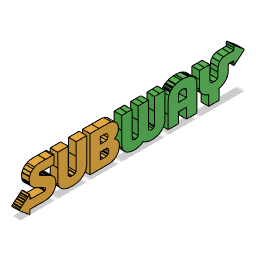
SUBWAY v0 (Autodesk Fusion 360 design; units mm, degrees)
Autodesk Fusion 360 part; units mm, degrees
note: some values were not read from the file. Set by a fixed rule: which sketch regions a step uses.
sketch "Sketch1" plane through (0, 0, 0) normal (1, 0, 0) x (0, 0, -1)
  spline S0 degree 3 poles (17.9669, -3.8504) (12.8198, -3.8249) (12.5225, -3.8587) (10.8168, -4.6775) knots 0 0 0 0 1 1 1 1
  spline S1 degree 3 poles (10.8168, -4.6775) (10.4326, -4.8619) (9.9837, -5.1092) (9.819, -5.2263) knots 0 0 0 0 1 1 1 1
  spline S2 degree 3 poles (9.819, -5.2263) (9.3261, -5.5771) (8.4224, -6.4653) (8.4224, -6.5991) knots 0 0 0 0 1 1 1 1
  spline S3 degree 3 poles (8.4224, -6.5991) (8.4224, -6.6674) (8.3955, -6.7231) (8.3627, -6.7231) knots 0 0 0 0 1 1 1 1
  spline S4 degree 3 poles (8.3627, -6.7231) (8.2047, -6.7231) (7.4935, -8.0577) (7.4922, -8.3563) knots 0 0 0 0 1 1 1 1
  spline S5 degree 3 poles (7.4922, -8.3563) (7.4918, -8.4679) (7.4655, -8.5874) (7.4341, -8.6222) knots 0 0 0 0 1 1 1 1
  spline S6 degree 3 poles (7.4341, -8.6222) (7.2242, -8.8543) (7.1579, -10.8776) (7.3318, -11.7452) knots 0 0 0 0 1 1 1 1
  spline S7 degree 3 poles (7.3318, -11.7452) (7.3904, -12.0379) (7.4649, -12.4116) (7.4977, -12.5762) knots 0 0 0 0 1 1 1 1
  spline S8 degree 3 poles (7.4977, -12.5762) (7.5599, -12.8888) (7.831, -13.454) (8.141, -13.9196) knots 0 0 0 0 1 1 1 1
  spline S9 degree 3 poles (8.141, -13.9196) (8.2411, -14.0697) (8.3527, -14.2401) (8.3891, -14.2986) knots 0 0 0 0 1 1 1 1
  spline S10 degree 3 poles (8.3891, -14.2986) (8.5537, -14.5634) (9.6552, -15.5795) (10.1208, -15.8954) knots 0 0 0 0 1 1 1 1
  spline S11 degree 3 poles (10.1208, -15.8954) (10.7697, -16.3356) (11.5575, -16.8141) (11.7594, -16.8915) knots 0 0 0 0 1 1 1 1
  spline S12 degree 3 poles (11.7594, -16.8915) (11.8446, -16.9241) (12.1837, -17.0969) (12.5129, -17.2752) knots 0 0 0 0 1 1 1 1
  spline S13 degree 3 poles (12.5129, -17.2752) (12.8421, -17.4534) (13.2458, -17.6552) (13.4105, -17.724) knots 0 0 0 0 1 1 1 1
  spline S14 degree 3 poles (13.4105, -17.724) (13.5751, -17.7928) (14.1293, -18.0504) (14.6414, -18.296) knots 0 0 0 0 1 1 1 1
  spline S15 degree 3 poles (14.6414, -18.296) (17.379, -19.6092) (17.6139, -19.7445) (17.8467, -20.1417) knots 0 0 0 0 1 1 1 1
  spline S16 degree 3 poles (17.8467, -20.1417) (18.0862, -20.5505) (18.0935, -20.9776) (17.8668, -21.3106) knots 0 0 0 0 1 1 1 1
  spline S17 degree 3 poles (17.8668, -21.3106) (17.7754, -21.4449) (17.6504, -21.5545) (17.5885, -21.5548) knots 0 0 0 0 1 1 1 1
  spline S18 degree 3 poles (17.5885, -21.5548) (17.5267, -21.555) (17.4543, -21.5906) (17.4281, -21.633) knots 0 0 0 0 1 1 1 1
  spline S19 degree 3 poles (17.4281, -21.633) (17.3789, -21.7122) (11.7353, -21.6755) (8.9377, -21.578) knots 0 0 0 0 1 1 1 1
  line L0 (8.9377, -21.578) -> (7.6905, -21.5346)
  line L1 (7.6905, -21.5346) -> (7.6905, -20.082)
  spline S20 degree 3 poles (7.6905, -20.082) (7.6905, -18.8349) (7.6762, -18.6286) (7.5905, -18.6286) knots 0 0 0 0 1 1 1 1
  spline S21 degree 3 poles (7.5905, -18.6286) (7.5357, -18.6286) (7.4913, -18.6586) (7.4913, -18.6952) knots 0 0 0 0 1 1 1 1
  spline S22 degree 3 poles (7.4913, -18.6952) (7.4913, -18.7318) (7.4571, -18.7619) (7.4153, -18.7619) knots 0 0 0 0 1 1 1 1
  spline S23 degree 3 poles (7.4153, -18.7619) (7.3328, -18.7619) (6.6268, -19.3372) (6.5402, -19.475) knots 0 0 0 0 1 1 1 1
  spline S24 degree 3 poles (6.5402, -19.475) (6.5109, -19.5216) (6.3962, -19.6068) (6.2852, -19.6642) knots 0 0 0 0 1 1 1 1
  spline S25 degree 3 poles (6.2852, -19.6642) (6.1742, -19.7216) (5.9129, -19.9253) (5.7054, -20.1161) knots 0 0 0 0 1 1 1 1
  spline S26 degree 3 poles (5.7054, -20.1161) (5.4978, -20.3069) (5.1889, -20.5586) (5.0186, -20.6758) knots 0 0 0 0 1 1 1 1
  spline S27 degree 3 poles (5.0186, -20.6758) (4.8483, -20.7929) (4.6992, -20.9123) (4.6868, -20.9409) knots 0 0 0 0 1 1 1 1
  spline S28 degree 3 poles (4.6868, -20.9409) (4.6532, -21.0188) (3.9986, -21.5555) (3.9372, -21.5555) knots 0 0 0 0 1 1 1 1
  spline S29 degree 3 poles (3.9372, -21.5555) (3.9079, -21.5555) (3.7899, -21.6549) (3.6752, -21.7765) knots 0 0 0 0 1 1 1 1
  spline S30 degree 3 poles (3.6752, -21.7765) (3.5602, -21.8987) (3.152, -22.2499) (2.7679, -22.5583) knots 0 0 0 0 1 1 1 1
  spline S31 degree 3 poles (2.7679, -22.5583) (2.3839, -22.8667) (2.0105, -23.179) (1.9378, -23.252) knots 0 0 0 0 1 1 1 1
  spline S32 degree 3 poles (1.9378, -23.252) (1.865, -23.3251) (1.6953, -23.4596) (1.561, -23.5513) knots 0 0 0 0 1 1 1 1
  spline S33 degree 3 poles (1.561, -23.5513) (1.4267, -23.6426) (1.1481, -23.8779) (0.9417, -24.0736) knots 0 0 0 0 1 1 1 1
  line L2 (0.9417, -24.0736) -> (0.5665, -24.4304)
  line L3 (0.5665, -24.4304) -> (0.9859, -24.8201)
  spline S34 degree 3 poles (0.9859, -24.8201) (1.2164, -25.0347) (1.4264, -25.2113) (1.4525, -25.2123) knots 0 0 0 0 1 1 1 1
  spline S35 degree 3 poles (1.4525, -25.2123) (1.4786, -25.2133) (1.7329, -25.4237) (2.0176, -25.6797) knots 0 0 0 0 1 1 1 1
  spline S36 degree 3 poles (2.0176, -25.6797) (2.3023, -25.9357) (2.5707, -26.1456) (2.6145, -26.1456) knots 0 0 0 0 1 1 1 1
  spline S37 degree 3 poles (2.6145, -26.1456) (2.6582, -26.1456) (2.7333, -26.1976) (2.7811, -26.2619) knots 0 0 0 0 1 1 1 1
  spline S38 degree 3 poles (2.7811, -26.2619) (2.8289, -26.3262) (3.0324, -26.5138) (3.233, -26.6782) knots 0 0 0 0 1 1 1 1
  spline S39 degree 3 poles (3.233, -26.6782) (3.4337, -26.8425) (3.6577, -27.0256) (3.7315, -27.0859) knots 0 0 0 0 1 1 1 1
  spline S40 degree 3 poles (3.7315, -27.0859) (3.8052, -27.1461) (4.0573, -27.3559) (4.2912, -27.5517) knots 0 0 0 0 1 1 1 1
  spline S41 degree 3 poles (4.2912, -27.5517) (4.525, -27.7475) (4.8442, -28.0037) (5.0004, -28.1207) knots 0 0 0 0 1 1 1 1
  spline S42 degree 3 poles (5.0004, -28.1207) (5.1566, -28.2376) (5.3877, -28.4367) (5.5143, -28.5633) knots 0 0 0 0 1 1 1 1
  spline S43 degree 3 poles (5.5143, -28.5633) (5.641, -28.6899) (5.8609, -28.8691) (6.0027, -28.9609) knots 0 0 0 0 1 1 1 1
  spline S44 degree 3 poles (6.0027, -28.9609) (6.1444, -29.0528) (6.4398, -29.2938) (6.6592, -29.4974) knots 0 0 0 0 1 1 1 1
  spline S45 degree 3 poles (6.6592, -29.4974) (6.8787, -29.7009) (7.0938, -29.8681) (7.1367, -29.8687) knots 0 0 0 0 1 1 1 1
  spline S46 degree 3 poles (7.1367, -29.8687) (7.1797, -29.8693) (7.2842, -29.9578) (7.3693, -30.0655) knots 0 0 0 0 1 1 1 1
  spline S47 degree 3 poles (7.3693, -30.0655) (7.6698, -30.446) (7.6865, -30.3812) (7.7057, -28.7555) knots 0 0 0 0 1 1 1 1
  line L4 (7.7057, -28.7555) -> (7.7235, -27.2425)
  line L5 (7.7235, -27.2425) -> (8.0227, -27.251)
  spline S48 degree 3 poles (8.0227, -27.251) (8.1873, -27.2553) (9.9156, -27.2648) (11.8635, -27.2727) knots 0 0 0 0 1 1 1 1
  spline S49 degree 3 poles (11.8635, -27.2727) (14.3296, -27.2827) (15.4052, -27.3091) (15.4052, -27.3587) knots 0 0 0 0 1 1 1 1
  spline S50 degree 3 poles (15.4052, -27.3587) (15.4052, -27.4401) (17.4754, -27.3847) (18.5314, -27.275) knots 0 0 0 0 1 1 1 1
  spline S51 degree 3 poles (18.5314, -27.275) (19.3597, -27.189) (20.4028, -26.9844) (20.5599, -26.8773) knots 0 0 0 0 1 1 1 1
  spline S52 degree 3 poles (20.5599, -26.8773) (20.5965, -26.8524) (20.8063, -26.7618) (21.0258, -26.6758) knots 0 0 0 0 1 1 1 1
  spline S53 degree 3 poles (21.0258, -26.6758) (21.2452, -26.5898) (21.44, -26.5011) (21.4583, -26.4789) knots 0 0 0 0 1 1 1 1
  spline S54 degree 3 poles (21.4583, -26.4789) (21.5226, -26.4008) (21.9988, -26.1448) (22.0799, -26.1448) knots 0 0 0 0 1 1 1 1
  spline S55 degree 3 poles (22.0799, -26.1448) (22.1251, -26.1448) (22.2664, -26.0482) (22.3939, -25.9293) knots 0 0 0 0 1 1 1 1
  spline S56 degree 3 poles (22.3939, -25.9293) (22.5214, -25.8104) (22.7399, -25.6228) (22.8799, -25.5131) knots 0 0 0 0 1 1 1 1
  spline S57 degree 3 poles (22.8799, -25.5131) (23.1681, -25.287) (23.8903, -24.3842) (24.1031, -23.9837) knots 0 0 0 0 1 1 1 1
  spline S58 degree 3 poles (24.1031, -23.9837) (24.3188, -23.5776) (24.6457, -22.5491) (24.7534, -21.9374) knots 0 0 0 0 1 1 1 1
  spline S59 degree 3 poles (24.7534, -21.9374) (24.969, -20.7123) (24.8306, -19.0957) (24.4255, -18.1027) knots 0 0 0 0 1 1 1 1
  spline S60 degree 3 poles (24.4255, -18.1027) (24.3297, -17.8678) (24.2511, -17.6501) (24.2511, -17.619) knots 0 0 0 0 1 1 1 1
  spline S61 degree 3 poles (24.2511, -17.619) (24.2511, -17.5505) (23.9224, -17.0259) (23.8209, -16.933) knots 0 0 0 0 1 1 1 1
  spline S62 degree 3 poles (23.8209, -16.933) (23.781, -16.8964) (23.6054, -16.68) (23.431, -16.4516) knots 0 0 0 0 1 1 1 1
  spline S63 degree 3 poles (23.431, -16.4516) (23.2566, -16.2233) (23.0527, -16.0038) (22.9783, -15.9641) knots 0 0 0 0 1 1 1 1
  spline S64 degree 3 poles (22.9783, -15.9641) (22.8475, -15.8941) (22.7341, -15.8017) (22.3094, -15.4238) knots 0 0 0 0 1 1 1 1
  spline S65 degree 3 poles (22.3094, -15.4238) (22.1989, -15.3254) (21.9991, -15.1942) (21.866, -15.1316) knots 0 0 0 0 1 1 1 1
  spline S66 degree 3 poles (21.866, -15.1316) (21.7329, -15.0689) (21.5204, -14.9319) (21.3932, -14.8277) knots 0 0 0 0 1 1 1 1
  spline S67 degree 3 poles (21.3932, -14.8277) (21.266, -14.7235) (21.1376, -14.6386) (21.1079, -14.6386) knots 0 0 0 0 1 1 1 1
  spline S68 degree 3 poles (21.1079, -14.6386) (21.0782, -14.6386) (20.8981, -14.5341) (20.708, -14.406) knots 0 0 0 0 1 1 1 1
  spline S69 degree 3 poles (20.708, -14.406) (20.5178, -14.278) (20.3211, -14.1727) (20.2708, -14.1727) knots 0 0 0 0 1 1 1 1
  spline S70 degree 3 poles (20.2708, -14.1727) (20.1639, -14.1727) (19.639, -13.8972) (19.6065, -13.8239) knots 0 0 0 0 1 1 1 1
  spline S71 degree 3 poles (19.6065, -13.8239) (19.5943, -13.7965) (19.542, -13.7743) (19.4902, -13.7743) knots 0 0 0 0 1 1 1 1
  spline S72 degree 3 poles (19.4902, -13.7743) (19.4384, -13.7743) (19.3964, -13.7442) (19.3964, -13.7076) knots 0 0 0 0 1 1 1 1
  spline S73 degree 3 poles (19.3964, -13.7076) (19.3964, -13.6711) (19.3473, -13.641) (19.2879, -13.641) knots 0 0 0 0 1 1 1 1
  spline S74 degree 3 poles (19.2879, -13.641) (19.2285, -13.641) (19.0116, -13.5562) (18.8058, -13.4526) knots 0 0 0 0 1 1 1 1
  spline S75 degree 3 poles (18.8058, -13.4526) (17.7171, -12.9047) (17.1625, -12.6389) (17.112, -12.641) knots 0 0 0 0 1 1 1 1
  spline S76 degree 3 poles (17.112, -12.641) (17.0811, -12.6424) (16.9742, -12.5854) (16.8749, -12.5147) knots 0 0 0 0 1 1 1 1
  spline S77 degree 3 poles (16.8749, -12.5147) (16.7755, -12.444) (16.6064, -12.3648) (16.4989, -12.3387) knots 0 0 0 0 1 1 1 1
  spline S78 degree 3 poles (16.4989, -12.3387) (16.3914, -12.3127) (15.9966, -12.1236) (15.6215, -11.9186) knots 0 0 0 0 1 1 1 1
  spline S79 degree 3 poles (15.6215, -11.9186) (15.2463, -11.7136) (14.8125, -11.4808) (14.6572, -11.4016) knots 0 0 0 0 1 1 1 1
  spline S80 degree 3 poles (14.6572, -11.4016) (14.5019, -11.3224) (14.2863, -11.1648) (14.1781, -11.0512) knots 0 0 0 0 1 1 1 1
  spline S81 degree 3 poles (14.1781, -11.0512) (13.9981, -10.8621) (13.9813, -10.8048) (13.9813, -10.3707) knots 0 0 0 0 1 1 1 1
  spline S82 degree 3 poles (13.9813, -10.3707) (13.9813, -9.9158) (13.9901, -9.8891) (14.2006, -9.7134) knots 0 0 0 0 1 1 1 1
  spline S83 degree 3 poles (14.2006, -9.7134) (14.3213, -9.6126) (14.5146, -9.5167) (14.63, -9.4994) knots 0 0 0 0 1 1 1 1
  spline S84 degree 3 poles (14.63, -9.4994) (14.7455, -9.4821) (16.8154, -9.4834) (19.2298, -9.5025) knots 0 0 0 0 1 1 1 1
  line L6 (19.2298, -9.5025) -> (23.6197, -9.5374)
  line L7 (23.6197, -9.5374) -> (23.6073, -6.75)
  line L8 (23.6073, -6.75) -> (23.5941, -3.9633)
  line L9 (23.5941, -3.9633) -> (22.8089, -3.9176)
  spline S85 degree 3 poles (22.8089, -3.9176) (22.3759, -3.8926) (20.1966, -3.8625) (17.9654, -3.8514) knots 0 0 0 0 1 1 1 1
  line L10 (17.9654, -3.8514) -> (17.9669, -3.8504)
  line L11 (26.1112, -3.8636) -> (26.1336, -12.8925)
  spline S86 degree 3 poles (26.1336, -12.8925) (26.1532, -20.9268) (26.1673, -21.9579) (26.2615, -22.254) knots 0 0 0 0 1 1 1 1
  spline S87 degree 3 poles (26.2615, -22.254) (26.459, -22.8741) (26.666, -23.3788) (26.8561, -23.7012) knots 0 0 0 0 1 1 1 1
  spline S88 degree 3 poles (26.8561, -23.7012) (26.9602, -23.8779) (27.046, -24.0519) (27.046, -24.088) knots 0 0 0 0 1 1 1 1
  spline S89 degree 3 poles (27.046, -24.088) (27.046, -24.3202) (28.785, -26.1452) (29.0063, -26.1452) knots 0 0 0 0 1 1 1 1
  spline S90 degree 3 poles (29.0063, -26.1452) (29.0305, -26.1452) (29.176, -26.2275) (29.3296, -26.3281) knots 0 0 0 0 1 1 1 1
  spline S91 degree 3 poles (29.3296, -26.3281) (30.0784, -26.8188) (30.3659, -26.9586) (31.1798, -27.2304) knots 0 0 0 0 1 1 1 1
  spline S92 degree 3 poles (31.1798, -27.2304) (32.073, -27.5287) (32.8887, -27.7261) (33.6967, -27.8389) knots 0 0 0 0 1 1 1 1
  spline S93 degree 3 poles (33.6967, -27.8389) (34.5621, -27.9597) (36.694, -27.961) (37.488, -27.8412) knots 0 0 0 0 1 1 1 1
  spline S94 degree 3 poles (37.488, -27.8412) (38.6521, -27.6656) (39.5088, -27.4479) (40.125, -27.1707) knots 0 0 0 0 1 1 1 1
  spline S95 degree 3 poles (40.125, -27.1707) (40.2403, -27.1188) (40.3853, -27.0761) (40.4467, -27.0761) knots 0 0 0 0 1 1 1 1
  spline S96 degree 3 poles (40.4467, -27.0761) (40.5792, -27.0761) (41.6532, -26.5137) (41.8443, -26.3444) knots 0 0 0 0 1 1 1 1
  spline S97 degree 3 poles (41.8443, -26.3444) (41.9174, -26.2796) (42.0873, -26.1708) (42.221, -26.1025) knots 0 0 0 0 1 1 1 1
  spline S98 degree 3 poles (42.221, -26.1025) (42.5395, -25.94) (43.6561, -24.904) (43.7883, -24.6483) knots 0 0 0 0 1 1 1 1
  spline S99 degree 3 poles (43.7883, -24.6483) (43.8451, -24.5386) (43.9561, -24.3839) (44.0348, -24.3042) knots 0 0 0 0 1 1 1 1
  spline S100 degree 3 poles (44.0348, -24.3042) (44.2262, -24.1106) (44.6826, -23.2713) (44.7829, -22.9283) knots 0 0 0 0 1 1 1 1
  spline S101 degree 3 poles (44.7829, -22.9283) (44.8271, -22.777) (44.9385, -22.3839) (45.0309, -22.0547) knots 0 0 0 0 1 1 1 1
  line L12 (45.0309, -22.0547) -> (45.1991, -21.4555)
  line L13 (45.1991, -21.4555) -> (45.2015, -12.6599)
  line L14 (45.2015, -12.6599) -> (45.2039, -3.8636)
  line L15 (45.2039, -3.8636) -> (41.7119, -3.8636)
  line L16 (41.7119, -3.8636) -> (38.2198, -3.8636)
  line L17 (38.2198, -3.8636) -> (38.2198, -12.2726)
  spline S102 degree 3 poles (38.2198, -12.2726) (38.2198, -17.4562) (38.1954, -20.7467) (38.1563, -20.8495) knots 0 0 0 0 1 1 1 1
  spline S103 degree 3 poles (38.1563, -20.8495) (38.0741, -21.0656) (37.6314, -21.5556) (37.5183, -21.5556) knots 0 0 0 0 1 1 1 1
  spline S104 degree 3 poles (37.5183, -21.5556) (37.4703, -21.5556) (37.3908, -21.5956) (37.3416, -21.6448) knots 0 0 0 0 1 1 1 1
  spline S105 degree 3 poles (37.3416, -21.6448) (37.1097, -21.8767) (36.5438, -21.9881) (35.5929, -21.9881) knots 0 0 0 0 1 1 1 1
  line L18 (35.5929, -21.9881) -> (34.6619, -21.9881)
  line L19 (34.6619, -21.9881) -> (34.1341, -21.7316)
  spline S106 degree 3 poles (34.1341, -21.7316) (33.5796, -21.4633) (33.4268, -21.3192) (33.1796, -20.8307) knots 0 0 0 0 1 1 1 1
  line L20 (33.1796, -20.8307) -> (33.03, -20.5353)
  line L21 (33.03, -20.5353) -> (33.03, -12.1994)
  line L22 (33.03, -12.1994) -> (33.03, -3.8634)
  line L23 (33.03, -3.8634) -> (29.5697, -3.8634)
  line L24 (29.5697, -3.8634) -> (26.1094, -3.8634)
  line L25 (26.1094, -3.8634) -> (26.1112, -3.8636)
  line L26 (47.3975, -3.8643) -> (47.3975, -15.6364)
  line L27 (47.3975, -15.6364) -> (47.3975, -27.4093)
  line L28 (47.3975, -27.4093) -> (53.6662, -27.407)
  spline S107 degree 3 poles (53.6662, -27.407) (60.04, -27.4049) (60.6452, -27.3851) (61.4306, -27.1473) knots 0 0 0 0 1 1 1 1
  spline S108 degree 3 poles (61.4306, -27.1473) (61.5584, -27.1087) (61.7446, -27.0768) (61.8446, -27.0768) knots 0 0 0 0 1 1 1 1
  spline S109 degree 3 poles (61.8446, -27.0768) (62.0206, -27.0768) (62.6478, -26.8233) (63.1933, -26.5319) knots 0 0 0 0 1 1 1 1
  spline S110 degree 3 poles (63.1933, -26.5319) (63.3397, -26.4537) (63.6234, -26.3022) (63.8235, -26.1955) knots 0 0 0 0 1 1 1 1
  spline S111 degree 3 poles (63.8235, -26.1955) (64.1353, -26.0291) (64.516, -25.7092) (65.1165, -25.1095) knots 0 0 0 0 1 1 1 1
  spline S112 degree 3 poles (65.1165, -25.1095) (65.2974, -24.9288) (65.7039, -24.3619) (65.9094, -24.0026) knots 0 0 0 0 1 1 1 1
  spline S113 degree 3 poles (65.9094, -24.0026) (66.0869, -23.6924) (66.489, -22.5389) (66.6233, -21.9554) knots 0 0 0 0 1 1 1 1
  spline S114 degree 3 poles (66.6233, -21.9554) (66.7371, -21.4609) (66.7969, -20.173) (66.7342, -19.561) knots 0 0 0 0 1 1 1 1
  spline S115 degree 3 poles (66.7342, -19.561) (66.6863, -19.0933) (66.4022, -18.0126) (66.2885, -17.865) knots 0 0 0 0 1 1 1 1
  spline S116 degree 3 poles (66.2885, -17.865) (66.2603, -17.8284) (66.199, -17.6788) (66.1528, -17.5324) knots 0 0 0 0 1 1 1 1
  spline S117 degree 3 poles (66.1528, -17.5324) (66.0268, -17.1328) (65.2329, -16.1727) (64.6661, -15.7349) knots 0 0 0 0 1 1 1 1
  spline S118 degree 3 poles (64.6661, -15.7349) (64.525, -15.6259) (64.3394, -15.4727) (64.2537, -15.3938) knots 0 0 0 0 1 1 1 1
  spline S119 degree 3 poles (64.2537, -15.3938) (64.168, -15.315) (63.9771, -15.1972) (63.8289, -15.1318) knots 0 0 0 0 1 1 1 1
  spline S120 degree 3 poles (63.8289, -15.1318) (63.6807, -15.0664) (63.5592, -14.994) (63.5592, -14.9714) knots 0 0 0 0 1 1 1 1
  spline S121 degree 3 poles (63.5592, -14.9714) (63.5592, -14.9304) (63.9281, -14.6388) (63.9801, -14.6388) knots 0 0 0 0 1 1 1 1
  spline S122 degree 3 poles (63.9801, -14.6388) (64.0297, -14.6388) (65.0893, -13.5925) (65.0893, -13.5435) knots 0 0 0 0 1 1 1 1
  spline S123 degree 3 poles (65.0893, -13.5435) (65.0893, -13.5171) (65.1453, -13.4158) (65.2141, -13.3187) knots 0 0 0 0 1 1 1 1
  spline S124 degree 3 poles (65.2141, -13.3187) (65.4108, -13.0414) (65.7945, -12.293) (65.8869, -12.0064) knots 0 0 0 0 1 1 1 1
  spline S125 degree 3 poles (65.8869, -12.0064) (65.9332, -11.8631) (66.0049, -11.7035) (66.0459, -11.6522) knots 0 0 0 0 1 1 1 1
  spline S126 degree 3 poles (66.0459, -11.6522) (66.0954, -11.5901) (66.118, -11.1331) (66.1148, -10.2887) knots 0 0 0 0 1 1 1 1
  spline S127 degree 3 poles (66.1148, -10.2887) (66.1103, -9.1063) (66.0981, -8.9805) (65.9342, -8.4648) knots 0 0 0 0 1 1 1 1
  spline S128 degree 3 poles (65.9342, -8.4648) (65.7321, -7.8289) (65.2664, -6.8576) (65.0226, -6.5634) knots 0 0 0 0 1 1 1 1
  spline S129 degree 3 poles (65.0226, -6.5634) (64.5939, -6.0458) (64.0884, -5.5515) (63.7096, -5.2805) knots 0 0 0 0 1 1 1 1
  spline S130 degree 3 poles (63.7096, -5.2805) (63.1831, -4.904) (62.2596, -4.4536) (61.5647, -4.2341) knots 0 0 0 0 1 1 1 1
  spline S131 degree 3 poles (61.5647, -4.2341) (60.4932, -3.8963) (59.7708, -3.8643) (53.3097, -3.8643) knots 0 0 0 0 1 1 1 1
  line L29 (53.3097, -3.8643) -> (47.3971, -3.8643)
  line L30 (47.3971, -3.8643) -> (47.3975, -3.8643)
  line L31 (54.2484, -8.9765) -> (56.1274, -8.9982)
  spline S132 degree 3 poles (56.1274, -8.9982) (58.1657, -9.0212) (58.1504, -9.0188) (58.6326, -9.4245) knots 0 0 0 0 1 1 1 1
  spline S133 degree 3 poles (58.6326, -9.4245) (59.1501, -9.86) (59.3525, -10.864) (59.1334, -11.9127) knots 0 0 0 0 1 1 1 1
  spline S134 degree 3 poles (59.1334, -11.9127) (59.0568, -12.2793) (58.6065, -12.8887) (58.2861, -13.0599) knots 0 0 0 0 1 1 1 1
  spline S135 degree 3 poles (58.2861, -13.0599) (58.0176, -13.2035) (57.9279, -13.2101) (56.1274, -13.2305) knots 0 0 0 0 1 1 1 1
  line L32 (56.1274, -13.2305) -> (54.2484, -13.2522)
  line L33 (54.2484, -13.2522) -> (54.2484, -11.1143)
  line L34 (54.2484, -11.1143) -> (54.2484, -8.9765)
  spline S136 degree 3 poles (54.298, -17.7526) (54.3255, -17.7413) (55.3082, -17.7467) (56.4816, -17.765) knots 0 0 0 0 1 1 1 1
  line L35 (56.4816, -17.765) -> (58.6148, -17.7983)
  line L36 (58.6148, -17.7983) -> (58.8946, -17.9836)
  spline S137 degree 3 poles (58.8946, -17.9836) (59.0487, -18.0856) (59.2857, -18.3405) (59.421, -18.5494) knots 0 0 0 0 1 1 1 1
  line L37 (59.421, -18.5494) -> (59.6667, -18.9293)
  line L38 (59.6667, -18.9293) -> (59.6675, -19.899)
  spline S138 degree 3 poles (59.6675, -19.899) (59.6683, -20.7868) (59.6553, -20.897) (59.5078, -21.2121) knots 0 0 0 0 1 1 1 1
  spline S139 degree 3 poles (59.5078, -21.2121) (59.4193, -21.4014) (59.3064, -21.5563) (59.2567, -21.5563) knots 0 0 0 0 1 1 1 1
  spline S140 degree 3 poles (59.2567, -21.5563) (59.2069, -21.5563) (59.1494, -21.599) (59.1295, -21.6508) knots 0 0 0 0 1 1 1 1
  spline S141 degree 3 poles (59.1295, -21.6508) (59.0721, -21.8004) (58.6328, -22.059) (58.2924, -22.1438) knots 0 0 0 0 1 1 1 1
  spline S142 degree 3 poles (58.2924, -22.1438) (58.0914, -22.1939) (57.3155, -22.2213) (56.1142, -22.2213) knots 0 0 0 0 1 1 1 1
  line L39 (56.1142, -22.2213) -> (54.2484, -22.2213)
  line L40 (54.2484, -22.2213) -> (54.2484, -19.9974)
  spline S143 degree 3 poles (54.2484, -19.9974) (54.2484, -18.7741) (54.2706, -17.7639) (54.298, -17.7526) knots 0 0 0 0 1 1 1 1
  spline S144 degree 3 poles (142.434, -0.8661) (142.3862, -0.8922) (142.3825, -1.191) (142.3813, -2.2505) knots 0 0 0 0 1 1 1 1
  line L41 (142.3813, -2.2505) -> (142.3797, -3.7302)
  line L42 (142.3797, -3.7302) -> (139.7032, -3.7318)
  spline S145 degree 3 poles (139.7032, -3.7318) (137.1275, -3.7331) (136.7848, -3.7522) (135.6459, -3.9558) knots 0 0 0 0 1 1 1 1
  spline S146 degree 3 poles (135.6459, -3.9558) (134.7048, -4.1241) (133.6691, -4.7468) (133.0438, -5.5209) knots 0 0 0 0 1 1 1 1
  spline S147 degree 3 poles (133.0438, -5.5209) (132.5335, -6.1524) (132.2214, -6.8603) (131.9702, -7.9541) knots 0 0 0 0 1 1 1 1
  spline S148 degree 3 poles (131.9702, -7.9541) (131.945, -8.0638) (131.9049, -9.3804) (131.881, -10.8802) knots 0 0 0 0 1 1 1 1
  spline S149 degree 3 poles (131.881, -10.8802) (131.8332, -13.8832) (131.8538, -13.7377) (131.3888, -14.3164) knots 0 0 0 0 1 1 1 1
  spline S150 degree 3 poles (131.3888, -14.3164) (131.012, -14.7855) (130.0923, -15.1032) (129.1107, -15.1032) knots 0 0 0 0 1 1 1 1
  spline S151 degree 3 poles (129.1107, -15.1032) (128.6308, -15.1032) (127.7928, -14.9093) (127.5077, -14.7327) knots 0 0 0 0 1 1 1 1
  spline S152 degree 3 poles (127.5077, -14.7327) (127.1453, -14.5083) (126.7397, -14.102) (126.6612, -13.8847) knots 0 0 0 0 1 1 1 1
  spline S153 degree 3 poles (126.6612, -13.8847) (126.6079, -13.7371) (126.575, -12.2087) (126.5511, -8.7848) knots 0 0 0 0 1 1 1 1
  line L43 (126.5511, -8.7848) -> (126.517, -3.8969)
  line L44 (126.517, -3.8969) -> (123.1079, -3.8799)
  line L45 (123.1079, -3.8799) -> (119.6996, -3.862)
  line L46 (119.6996, -3.862) -> (119.7004, -9.0671)
  spline S154 degree 3 poles (119.7004, -9.0671) (119.7012, -11.9299) (119.729, -14.4618) (119.7624, -14.6932) knots 0 0 0 0 1 1 1 1
  spline S155 degree 3 poles (119.7624, -14.6932) (119.8358, -15.2002) (120.1152, -16.144) (120.3275, -16.6008) knots 0 0 0 0 1 1 1 1
  spline S156 degree 3 poles (120.3275, -16.6008) (120.7281, -17.4629) (121.6691, -18.5402) (122.5336, -19.1278) knots 0 0 0 0 1 1 1 1
  spline S157 degree 3 poles (122.5336, -19.1278) (122.7489, -19.2741) (122.9843, -19.4476) (123.0568, -19.513) knots 0 0 0 0 1 1 1 1
  spline S158 degree 3 poles (123.0568, -19.513) (123.1293, -19.5784) (123.2638, -19.6492) (123.356, -19.6704) knots 0 0 0 0 1 1 1 1
  spline S159 degree 3 poles (123.356, -19.6704) (123.4482, -19.6916) (123.6455, -19.7783) (123.7948, -19.8634) knots 0 0 0 0 1 1 1 1
  spline S160 degree 3 poles (123.7948, -19.8634) (124.1062, -20.0408) (124.9715, -20.3949) (125.4358, -20.5346) knots 0 0 0 0 1 1 1 1
  line L47 (125.4358, -20.5346) -> (125.752, -20.63)
  line L48 (125.752, -20.63) -> (125.752, -24.0189)
  line L49 (125.752, -24.0189) -> (125.752, -27.4087)
  line L50 (125.752, -27.4087) -> (129.2107, -27.4087)
  line L51 (129.2107, -27.4087) -> (132.6694, -27.4087)
  line L52 (132.6694, -27.4087) -> (132.6694, -24.0321)
  line L53 (132.6694, -24.0321) -> (132.6694, -20.6556)
  line L54 (132.6694, -20.6556) -> (133.2182, -20.4657)
  spline S161 degree 3 poles (133.2182, -20.4657) (134.0185, -20.1889) (135.572, -19.4134) (135.9901, -19.082) knots 0 0 0 0 1 1 1 1
  spline S162 degree 3 poles (135.9901, -19.082) (136.5198, -18.6623) (137.3717, -17.7807) (137.6172, -17.3984) knots 0 0 0 0 1 1 1 1
  spline S163 degree 3 poles (137.6172, -17.3984) (137.9206, -16.9259) (138.3516, -15.944) (138.4784, -15.4365) knots 0 0 0 0 1 1 1 1
  spline S164 degree 3 poles (138.4784, -15.4365) (138.6593, -14.7121) (138.7198, -13.8269) (138.7217, -11.8453) knots 0 0 0 0 1 1 1 1
  spline S165 degree 3 poles (138.7217, -11.8453) (138.7229, -10.8027) (138.7416, -9.8824) (138.7636, -9.8005) knots 0 0 0 0 1 1 1 1
  spline S166 degree 3 poles (138.7636, -9.8005) (138.8286, -9.5579) (139.1739, -9.5127) (140.8286, -9.5323) knots 0 0 0 0 1 1 1 1
  line L55 (140.8286, -9.5323) -> (142.3463, -9.5501)
  line L56 (142.3463, -9.5501) -> (142.3649, -10.9973)
  spline S167 degree 3 poles (142.3649, -10.9973) (142.376, -11.886) (142.4078, -12.4437) (142.4479, -12.4437) knots 0 0 0 0 1 1 1 1
  spline S168 degree 3 poles (142.4479, -12.4437) (142.4837, -12.4437) (142.513, -12.4136) (142.513, -12.377) knots 0 0 0 0 1 1 1 1
  spline S169 degree 3 poles (142.513, -12.377) (142.513, -12.3405) (142.5502, -12.3105) (142.5959, -12.3104) knots 0 0 0 0 1 1 1 1
  spline S170 degree 3 poles (142.5959, -12.3104) (142.6417, -12.3102) (142.9087, -12.1004) (143.1889, -11.8445) knots 0 0 0 0 1 1 1 1
  spline S171 degree 3 poles (143.1889, -11.8445) (143.4692, -11.5886) (143.7239, -11.3794) (143.7555, -11.3794) knots 0 0 0 0 1 1 1 1
  spline S172 degree 3 poles (143.7555, -11.3794) (143.7871, -11.3794) (143.9918, -11.2104) (144.2097, -11.0042) knots 0 0 0 0 1 1 1 1
  spline S173 degree 3 poles (144.2097, -11.0042) (144.4277, -10.7981) (144.7113, -10.5615) (144.8399, -10.4779) knots 0 0 0 0 1 1 1 1
  spline S174 degree 3 poles (144.8399, -10.4779) (144.9686, -10.3944) (145.253, -10.159) (145.4725, -9.9555) knots 0 0 0 0 1 1 1 1
  spline S175 degree 3 poles (145.4725, -9.9555) (145.692, -9.7519) (145.8942, -9.5855) (145.9213, -9.5849) knots 0 0 0 0 1 1 1 1
  spline S176 degree 3 poles (145.9213, -9.5849) (145.9484, -9.5844) (146.1297, -9.4417) (146.3244, -9.2679) knots 0 0 0 0 1 1 1 1
  spline S177 degree 3 poles (146.3244, -9.2679) (146.7573, -8.8814) (148.023, -7.8299) (148.394, -7.5486) knots 0 0 0 0 1 1 1 1
  spline S178 degree 3 poles (148.394, -7.5486) (148.5433, -7.4354) (148.83, -7.1874) (149.0312, -6.9975) knots 0 0 0 0 1 1 1 1
  line L57 (149.0312, -6.9975) -> (149.397, -6.6518)
  line L58 (149.397, -6.6518) -> (148.9405, -6.2224)
  spline S179 degree 3 poles (148.9405, -6.2224) (148.6894, -5.9859) (148.4444, -5.7922) (148.3963, -5.7922) knots 0 0 0 0 1 1 1 1
  spline S180 degree 3 poles (148.3963, -5.7922) (148.3483, -5.7922) (148.2545, -5.7241) (148.1878, -5.641) knots 0 0 0 0 1 1 1 1
  spline S181 degree 3 poles (148.1878, -5.641) (148.1211, -5.5579) (147.8872, -5.3489) (147.6677, -5.1759) knots 0 0 0 0 1 1 1 1
  spline S182 degree 3 poles (147.6677, -5.1759) (147.4482, -5.003) (147.2084, -4.8056) (147.1352, -4.7372) knots 0 0 0 0 1 1 1 1
  spline S183 degree 3 poles (147.1352, -4.7372) (147.062, -4.6688) (146.6816, -4.3531) (146.2895, -4.0357) knots 0 0 0 0 1 1 1 1
  spline S184 degree 3 poles (146.2895, -4.0357) (145.8974, -3.7182) (145.4883, -3.3701) (145.3803, -3.2621) knots 0 0 0 0 1 1 1 1
  spline S185 degree 3 poles (145.3803, -3.2621) (145.2722, -3.154) (145.157, -3.0652) (145.1245, -3.0652) knots 0 0 0 0 1 1 1 1
  spline S186 degree 3 poles (145.1245, -3.0652) (145.0919, -3.0652) (144.8381, -2.8562) (144.5601, -2.6001) knots 0 0 0 0 1 1 1 1
  spline S187 degree 3 poles (144.5601, -2.6001) (144.2823, -2.3452) (144.0244, -2.1354) (143.9926, -2.1354) knots 0 0 0 0 1 1 1 1
  spline S188 degree 3 poles (143.9926, -2.1354) (143.9586, -2.1354) (143.7538, -1.9692) (143.5376, -1.7656) knots 0 0 0 0 1 1 1 1
  spline S189 degree 3 poles (143.5376, -1.7656) (143.3214, -1.5621) (143.025, -1.3187) (142.8787, -1.2254) knots 0 0 0 0 1 1 1 1
  spline S190 degree 3 poles (142.8787, -1.2254) (142.7324, -1.1321) (142.5605, -0.9919) (142.4973, -0.9138) knots 0 0 0 0 1 1 1 1
  spline S191 degree 3 poles (142.4973, -0.9138) (142.4699, -0.8799) (142.4497, -0.8585) (142.4338, -0.8672) knots 0 0 0 0 1 1 1 1
  line L59 (142.4338, -0.8672) -> (142.434, -0.8661)
  spline S192 degree 3 poles (108.6973, -3.1613) (108.2854, -3.1547) (107.8754, -3.1666) (107.4756, -3.1977) knots 0 0 0 0 1 1 1 1
  spline S193 degree 3 poles (107.4756, -3.1977) (106.1692, -3.2995) (104.8711, -3.5671) (104.1208, -3.8899) knots 0 0 0 0 1 1 1 1
  spline S194 degree 3 poles (104.1208, -3.8899) (103.9848, -3.9484) (103.8228, -3.9969) (103.7604, -3.9969) knots 0 0 0 0 1 1 1 1
  spline S195 degree 3 poles (103.7604, -3.9969) (103.6164, -3.9969) (102.6676, -4.4828) (102.3186, -4.7356) knots 0 0 0 0 1 1 1 1
  spline S196 degree 3 poles (102.3186, -4.7356) (102.173, -4.8411) (102.0174, -4.9278) (101.9737, -4.9278) knots 0 0 0 0 1 1 1 1
  spline S197 degree 3 poles (101.9737, -4.9278) (101.9299, -4.9278) (101.7928, -5.0249) (101.6683, -5.1441) knots 0 0 0 0 1 1 1 1
  spline S198 degree 3 poles (101.6683, -5.1441) (101.5438, -5.2632) (101.2543, -5.5227) (101.0257, -5.72) knots 0 0 0 0 1 1 1 1
  spline S199 degree 3 poles (101.0257, -5.72) (100.797, -5.9173) (100.6102, -6.1073) (100.6102, -6.1425) knots 0 0 0 0 1 1 1 1
  spline S200 degree 3 poles (100.6102, -6.1425) (100.6102, -6.1777) (100.4952, -6.3449) (100.3544, -6.5146) knots 0 0 0 0 1 1 1 1
  spline S201 degree 3 poles (100.3544, -6.5146) (99.9248, -7.0323) (99.7634, -7.3253) (99.487, -8.0873) knots 0 0 0 0 1 1 1 1
  spline S202 degree 3 poles (99.487, -8.0873) (98.9898, -9.4582) (99.0142, -8.9124) (99.0142, -18.6696) knots 0 0 0 0 1 1 1 1
  line L60 (99.0142, -18.6696) -> (99.0142, -27.4088)
  line L61 (99.0142, -27.4088) -> (102.4396, -27.4088)
  line L62 (102.4396, -27.4088) -> (105.8642, -27.4088)
  line L63 (105.8642, -27.4088) -> (105.8642, -24.0168)
  line L64 (105.8642, -24.0168) -> (105.8642, -20.6247)
  line L65 (105.8642, -20.6247) -> (108.4919, -20.6247)
  line L66 (108.4919, -20.6247) -> (111.1189, -20.6247)
  line L67 (111.1189, -20.6247) -> (111.1189, -24.0168)
  line L68 (111.1189, -24.0168) -> (111.1189, -27.4088)
  line L69 (111.1189, -27.4088) -> (114.5443, -27.4088)
  line L70 (114.5443, -27.4088) -> (117.9696, -27.4088)
  line L71 (117.9696, -27.4088) -> (117.9696, -18.7125)
  spline S203 degree 3 poles (117.9696, -18.7125) (117.9695, -11.1679) (117.9557, -9.9384) (117.8665, -9.4284) knots 0 0 0 0 1 1 1 1
  spline S204 degree 3 poles (117.8665, -9.4284) (117.7078, -8.5209) (117.1613, -7.1123) (116.8449, -6.796) knots 0 0 0 0 1 1 1 1
  spline S205 degree 3 poles (116.8449, -6.796) (116.7772, -6.7283) (116.6006, -6.4944) (116.4527, -6.2766) knots 0 0 0 0 1 1 1 1
  spline S206 degree 3 poles (116.4527, -6.2766) (116.3048, -6.0589) (116.1132, -5.8344) (116.0264, -5.7775) knots 0 0 0 0 1 1 1 1
  spline S207 degree 3 poles (116.0264, -5.7775) (115.9395, -5.7206) (115.7073, -5.5212) (115.5109, -5.3349) knots 0 0 0 0 1 1 1 1
  spline S208 degree 3 poles (115.5109, -5.3349) (115.3145, -5.1485) (115.094, -4.9774) (115.021, -4.9543) knots 0 0 0 0 1 1 1 1
  spline S209 degree 3 poles (115.021, -4.9543) (114.948, -4.9311) (114.7516, -4.814) (114.5838, -4.6946) knots 0 0 0 0 1 1 1 1
  spline S210 degree 3 poles (114.5838, -4.6946) (114.1949, -4.4169) (113.5122, -4.0749) (113.1233, -3.9614) knots 0 0 0 0 1 1 1 1
  spline S211 degree 3 poles (113.1233, -3.9614) (112.9566, -3.9127) (112.5637, -3.7936) (112.2542, -3.697) knots 0 0 0 0 1 1 1 1
  spline S212 degree 3 poles (112.2542, -3.697) (111.1905, -3.367) (109.9364, -3.1812) (108.7021, -3.1614) knots 0 0 0 0 1 1 1 1
  line L72 (108.7021, -3.1614) -> (108.6973, -3.1613)
  line L73 (96.8902, -3.862) -> (93.4463, -3.8798)
  line L74 (93.4463, -3.8798) -> (90.0015, -3.8969)
  line L75 (90.0015, -3.8969) -> (89.9682, -12.3436)
  line L76 (89.9682, -12.3436) -> (89.9348, -20.7911)
  line L77 (89.9348, -20.7911) -> (89.7558, -21.0949)
  spline S213 degree 3 poles (89.7558, -21.0949) (89.5334, -21.4731) (89.496, -21.5032) (89.0039, -21.6871) knots 0 0 0 0 1 1 1 1
  spline S214 degree 3 poles (89.0039, -21.6871) (88.2185, -21.9807) (86.9259, -21.8388) (86.4568, -21.4073) knots 0 0 0 0 1 1 1 1
  spline S215 degree 3 poles (86.4568, -21.4073) (86.3666, -21.3244) (86.2375, -21.1366) (86.1699, -20.9903) knots 0 0 0 0 1 1 1 1
  spline S216 degree 3 poles (86.1699, -20.9903) (86.0526, -20.7362) (86.0475, -20.35) (86.0459, -12.3987) knots 0 0 0 0 1 1 1 1
  spline S217 degree 3 poles (86.0459, -12.3987) (86.0451, -7.82) (86.0263, -4.027) (86.0041, -3.9691) knots 0 0 0 0 1 1 1 1
  spline S218 degree 3 poles (86.0041, -3.9691) (85.968, -3.8751) (85.604, -3.8637) (82.5787, -3.8637) knots 0 0 0 0 1 1 1 1
  line L78 (82.5787, -3.8637) -> (79.1936, -3.8637)
  line L79 (79.1936, -3.8637) -> (79.1936, -12.1949)
  spline S219 degree 3 poles (79.1936, -12.1949) (79.1936, -17.3943) (79.1689, -20.611) (79.1285, -20.7519) knots 0 0 0 0 1 1 1 1
  spline S220 degree 3 poles (79.1285, -20.7519) (78.9584, -21.3452) (78.4208, -21.7212) (77.593, -21.8262) knots 0 0 0 0 1 1 1 1
  spline S221 degree 3 poles (77.593, -21.8262) (77.0948, -21.8895) (76.4332, -21.8154) (76.124, -21.6611) knots 0 0 0 0 1 1 1 1
  spline S222 degree 3 poles (76.124, -21.6611) (76.0084, -21.6035) (75.8786, -21.5565) (75.8357, -21.5565) knots 0 0 0 0 1 1 1 1
  spline S223 degree 3 poles (75.8357, -21.5565) (75.7145, -21.5565) (75.502, -21.2865) (75.3628, -20.9573) knots 0 0 0 0 1 1 1 1
  spline S224 degree 3 poles (75.3628, -20.9573) (75.2411, -20.6693) (75.2356, -20.3452) (75.2194, -12.3439) knots 0 0 0 0 1 1 1 1
  spline S225 degree 3 poles (75.2194, -12.3439) (75.2102, -7.7711) (75.2023, -3.9933) (75.2024, -3.9476) knots 0 0 0 0 1 1 1 1
  spline S226 degree 3 poles (75.2024, -3.9476) (75.2025, -3.8822) (74.473, -3.8639) (71.777, -3.8639) knots 0 0 0 0 1 1 1 1
  line L80 (71.777, -3.8639) -> (68.3516, -3.8639)
  line L81 (68.3516, -3.8639) -> (68.3516, -12.5023)
  spline S227 degree 3 poles (68.3516, -12.5023) (68.3516, -22.0019) (68.339, -21.6614) (68.7625, -22.9528) knots 0 0 0 0 1 1 1 1
  spline S228 degree 3 poles (68.7625, -22.9528) (69.1268, -24.0639) (69.5949, -24.807) (70.4554, -25.6379) knots 0 0 0 0 1 1 1 1
  spline S229 degree 3 poles (70.4554, -25.6379) (70.7435, -25.9161) (71, -26.1443) (71.0251, -26.1448) knots 0 0 0 0 1 1 1 1
  spline S230 degree 3 poles (71.0251, -26.1448) (71.0502, -26.1454) (71.2636, -26.2779) (71.4995, -26.4394) knots 0 0 0 0 1 1 1 1
  spline S231 degree 3 poles (71.4995, -26.4394) (72.0737, -26.8326) (72.1922, -26.8894) (73.025, -27.1704) knots 0 0 0 0 1 1 1 1
  spline S232 degree 3 poles (73.025, -27.1704) (73.867, -27.4544) (74.4278, -27.593) (75.2024, -27.7091) knots 0 0 0 0 1 1 1 1
  line L82 (75.2024, -27.7091) -> (75.2032, -27.7091)
  spline S233 degree 3 poles (75.2032, -27.7091) (76.0131, -27.8305) (77.8365, -27.8299) (78.5316, -27.7083) knots 0 0 0 0 1 1 1 1
  spline S234 degree 3 poles (78.5316, -27.7083) (79.3642, -27.5626) (80.7832, -27.1096) (81.2478, -26.8409) knots 0 0 0 0 1 1 1 1
  spline S235 degree 3 poles (81.2478, -26.8409) (81.3714, -26.7694) (81.6105, -26.6158) (81.7795, -26.4991) knots 0 0 0 0 1 1 1 1
  spline S236 degree 3 poles (81.7795, -26.4991) (82.3906, -26.077) (82.5681, -26.0013) (82.7345, -26.0945) knots 0 0 0 0 1 1 1 1
  spline S237 degree 3 poles (82.7345, -26.0945) (82.8171, -26.1407) (82.8999, -26.1971) (82.9182, -26.2193) knots 0 0 0 0 1 1 1 1
  spline S238 degree 3 poles (82.9182, -26.2193) (82.9997, -26.3179) (84.2323, -27.0178) (84.3816, -27.0502) knots 0 0 0 0 1 1 1 1
  spline S239 degree 3 poles (84.3816, -27.0502) (84.4731, -27.0701) (84.6227, -27.1178) (84.7142, -27.1564) knots 0 0 0 0 1 1 1 1
  spline S240 degree 3 poles (84.7142, -27.1564) (85.0735, -27.3081) (85.8388, -27.5363) (86.3769, -27.6525) knots 0 0 0 0 1 1 1 1
  spline S241 degree 3 poles (86.3769, -27.6525) (87.1788, -27.8258) (89.5374, -27.8273) (90.4008, -27.6549) knots 0 0 0 0 1 1 1 1
  spline S242 degree 3 poles (90.4008, -27.6549) (91.0356, -27.528) (91.7995, -27.3183) (92.1301, -27.1805) knots 0 0 0 0 1 1 1 1
  spline S243 degree 3 poles (92.1301, -27.1805) (92.2399, -27.1347) (92.4497, -27.0598) (92.596, -27.0138) knots 0 0 0 0 1 1 1 1
  spline S244 degree 3 poles (92.596, -27.0138) (92.7423, -26.9678) (92.9664, -26.863) (93.0944, -26.7813) knots 0 0 0 0 1 1 1 1
  spline S245 degree 3 poles (93.0944, -26.7813) (93.2224, -26.6995) (93.5358, -26.5008) (93.7904, -26.3394) knots 0 0 0 0 1 1 1 1
  spline S246 degree 3 poles (93.7904, -26.3394) (94.0451, -26.1781) (94.4686, -25.8366) (94.7315, -25.5806) knots 0 0 0 0 1 1 1 1
  spline S247 degree 3 poles (94.7315, -25.5806) (95.2653, -25.0606) (95.9542, -24.1834) (95.9554, -24.0225) knots 0 0 0 0 1 1 1 1
  spline S248 degree 3 poles (95.9554, -24.0225) (95.9558, -23.9648) (96.0312, -23.786) (96.1229, -23.6256) knots 0 0 0 0 1 1 1 1
  spline S249 degree 3 poles (96.1229, -23.6256) (96.3172, -23.2856) (96.5679, -22.5823) (96.7298, -21.9219) knots 0 0 0 0 1 1 1 1
  spline S250 degree 3 poles (96.7298, -21.9219) (96.8341, -21.4962) (96.8457, -20.6976) (96.867, -12.6596) knots 0 0 0 0 1 1 1 1
  line L83 (96.867, -12.6596) -> (96.8903, -3.8625)
  line L84 (96.8903, -3.8625) -> (96.8902, -3.862)
  spline S251 degree 3 poles (108.1801, -9.0627) (108.3544, -9.0561) (108.5448, -9.057) (108.7576, -9.065) knots 0 0 0 0 1 1 1 1
  spline S252 degree 3 poles (108.7576, -9.065) (109.414, -9.0896) (109.541, -9.1153) (109.9886, -9.3169) knots 0 0 0 0 1 1 1 1
  spline S253 degree 3 poles (109.9886, -9.3169) (110.6445, -9.6124) (110.744, -9.7107) (110.9474, -10.2595) knots 0 0 0 0 1 1 1 1
  line L85 (110.9474, -10.2595) -> (111.1187, -10.7223)
  line L86 (111.1187, -10.7223) -> (111.1187, -12.9461)
  line L87 (111.1187, -12.9461) -> (111.1187, -15.1708)
  line L88 (111.1187, -15.1708) -> (108.4894, -15.1708)
  line L89 (108.4894, -15.1708) -> (105.8601, -15.1708)
  line L90 (105.8601, -15.1708) -> (105.8787, -12.826)
  line L91 (105.8787, -12.826) -> (105.8981, -10.482)
  line L92 (105.8981, -10.482) -> (106.0764, -10.1138)
  spline S254 degree 3 poles (106.0764, -10.1138) (106.2887, -9.6754) (106.378, -9.5914) (106.8802, -9.358) knots 0 0 0 0 1 1 1 1
  spline S255 degree 3 poles (106.8802, -9.358) (107.2807, -9.1719) (107.6574, -9.0825) (108.1801, -9.0627) knots 0 0 0 0 1 1 1 1
extrude "Extrude1" add sketch "Sketch1" against normal blind 5 makes body 1 at (0, -9.6277, -93.4271) makes body 2 at (0, -23.5075, -11.6716) makes body 3 at (0, -14.4372, -115.6516) makes body 4 at (0, -14.842, -49.6812) makes body 5 at (0, -12.4304, -30.7312) makes body 6 at (0, -22.8981, -128.0578)
